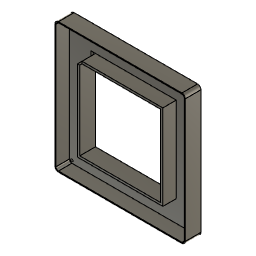
Macro Keyboard Base v2 (Autodesk Fusion 360 design; units mm, degrees)
Autodesk Fusion 360 part; units mm, degrees
sketch "Sketch1" plane through (0, 0, 0) normal (0, 1, 0) x (1, 0, 0)
  line L0 (-5, 8) -> (105, 8)
  line L1 (-8, -105) -> (-8, 5)
  line L2 (108, 5) -> (108, -105)
  line L3 (105, -108) -> (-5, -108)
  circle A0 centre (-5, 5) radius 1.1
  circle A1 centre (105, -105) radius 1.1
  arc A2 (105, -108) -> (108, -105) centre (105, -105) ccw
  arc A3 (-5, 8) -> (-8, 5) centre (-5, 5) ccw
  circle A4 centre (105, 5) radius 1.1
  arc A5 (-8, -105) -> (-5, -108) centre (-5, -105) ccw
  circle A6 centre (-5, -105) radius 1.1
  arc A7 (108, 5) -> (105, 8) centre (105, 5) ccw
  line L4 (-7.2, -105) -> (-7.2, 5)
  arc A8 (-5, 7.2) -> (-7.2, 5) centre (-5, 5) ccw
  line L5 (-5, 7.2) -> (105, 7.2)
  arc A9 (107.2, 5) -> (105, 7.2) centre (105, 5) ccw
  line L6 (107.2, 5) -> (107.2, -105)
  arc A10 (105, -107.2) -> (107.2, -105) centre (105, -105) ccw
  line L7 (105, -107.2) -> (-5, -107.2)
  arc A11 (-7.2, -105) -> (-5, -107.2) centre (-5, -105) ccw
  line L8 (88, -88) -> (12, -88)
  line L9 (12, -88) -> (12, -12)
  line L10 (12, -12) -> (88, -12)
  line L11 (88, -12) -> (88, -88)
  line L12 (86, -86) -> (14, -86)
  line L13 (14, -86) -> (14, -14)
  line L14 (14, -14) -> (86, -14)
  line L15 (86, -14) -> (86, -86)
  dimension "d27" = 2.2
  dimension "d28" = 2.2
  dimension "d29" = 2.2
  dimension "d30" = 2.2
  dimension "d35" = 3
  dimension "d36" = 3
  dimension "d37" = 3
  dimension "d38" = 3
  dimension "d43" = 0.8
  dimension "d67" = 20
  dimension "d68" = 22
  constraint tangent L0 A3
  constraint tangent L1 A3
  constraint tangent L0 A7
  constraint tangent L2 A7
  constraint tangent L3 A2
  constraint tangent L2 A2
  constraint tangent L1 A5
  constraint tangent L3 A5
  measures "d27" diameter of A1
  measures "d28" diameter of A4
  measures "d29" diameter of A0
  measures "d30" diameter of A6
  measures "d35" radius of A3
  measures "d36" radius of A7
  measures "d37" radius of A2
  measures "d38" radius of A5
extrude "Extrude1" add sketch "Sketch1" along normal blind 2 contours L0 L1 L2 L3 A2 A3 A5 A7 | L4 A8 L5 A9 L6 A10 L7 A11 | L8 L9 L10 L11 | L12 L13 L14 L15
extrude "Extrude2" add sketch "Sketch1" against normal blind 2 contours L0 L1 L2 L3 A2 A3 A5 A7
extrude "Extrude4" add 1 faces at (-7.4667, -2, 68.3333) along direction (0, -1, 0) blind 8
extrude "Extrude7" add 1 faces at (-7.4667, -10, 68.3333) along direction (0, -1, 0) blind 2
extrude "Extrude9" cut sketch "Sketch1" along normal blind 10 contours L12 L13 L14 L15
extrude "Extrude10" add sketch "Sketch1" against normal up to surface (12 mm away) contours L8 L9 L10 L11
sketch "Sketch4" plane through (0, -12, 0) normal (0, -1, 0) x (1, 0, 0)
  line L0 (86, 86) -> (86, 14)
  line L1 (86, 14) -> (14, 14)
  line L2 (14, 14) -> (14, 86)
  line L3 (14, 86) -> (86, 86)
  line L4 (12, 88) -> (12, 12)
  line L5 (12, 12) -> (88, 12)
  line L6 (88, 12) -> (88, 88)
  line L7 (88, 88) -> (12, 88)
  line L8 (12, 88) -> (16, 88)
  line L9 (16, 88) -> (16, 84)
  line L10 (16, 84) -> (12, 84)
  line L11 (12, 84) -> (12, 88)
  dimension "d73" = 4
  dimension "d74" = 4
  constraint horizontal L8
  constraint vertical L9
  constraint horizontal L10
  constraint vertical L11
  constraint coincident L4.start L7.end
  measures "d73" distance of L4.start L8.end
  measures "d74" distance of L4.start L10.end
extrude "Extrude11" cut sketch "Sketch4" against normal blind 47 contours L2 L3 L4 L7 L8 L9 L10 L11
